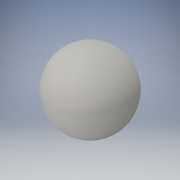
# Autodesk Inventor part: bearing sumo jeffrey p
Saved by Autodesk Inventor 2016 (Build 200138000, 138)
## iProperties
Created: 2017-09-07
Part Number: bearing sumo jeffrey p
Material: Generic
Document SubType Name: Modeling
Designer: student
Density: 1 g/cm^3
Appearance: Default
Author: student
Autodesk Inventor part; units mm, degrees
ref_plane "YZ Plane" through (0, 0, 0) normal (1, 0, 0) x (0, 1, 0)
ref_plane "XZ Plane" through (0, 0, 0) normal (0, 1, 0) x (-1, 0, 0)
ref_plane "XY Plane" through (0, 0, 0) normal (0, 0, 1) x (1, 0, 0)
sketch "Sketch1" plane through (0, 0, 0) normal (0, 0, 1) x (1, 0, 0)
  line L0 (0, 0) -> (0, 15.24)
  arc A0 (0, 8.7518) -> (0, -8.7518) centre (0, 0) ccw
  line L1 (0, -8.7518) -> (0, -7.8064)
  line L2 (0, 8.7518) -> (0, 7.62)
  arc A1 (0, 7.62) -> (0, -7.8064) centre (-0.2878, -0.0932) ccw
  dimension "d0" = 15.24
  dimension "d1" = 0.0932
  constraints: 6 end point, 4 point on circle, 2 centre point, 2 vertical, 1 coincident, 1 midpoint, 1 point on line
  measures "d0" distance of L0.start L0.end
  measures "d1" vertical distance of A0.centre A1.centre
revolve "Revolution1" add sketch "Sketch1" angle 360 about axis through (0, 0, 0) along (0, 1, 0)
body "Solid1"
